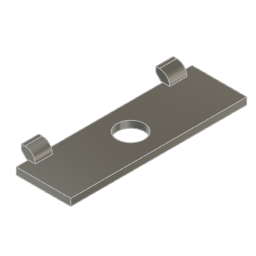
Mouse_ReplacementDoor (Autodesk Fusion 360 design; units mm, degrees)
Autodesk Fusion 360 part; units mm, degrees
sketch "Sketch1" plane through (0, 0, 0) normal (0, 0, 1) x (1, 0, 0)
  line L0 (0, 0) -> (15.8, 0)
  line L1 (15.8, 0) -> (15.8, 51)
  line L2 (15.8, 51) -> (0, 51)
  line L3 (0, 51) -> (0, 0)
  dimension "d1" = 15.8
  dimension "d2" = 51
  constraint horizontal L0
  constraint vertical L1
  constraint horizontal L2
  constraint vertical L3
  constraint coincident L0.start L3.end
  measures "d1" distance of L1.end L2.end
  measures "d2" distance of L0.end L1.end
extrude "Extrude1" add sketch "Sketch1" along normal blind 2
sketch "Sketch2" plane through (0, 0, 0) normal (0, 0, -1) x (1, 0, 0)
  line L0 (0, 0) -> (0, -51)
  line L1 (0, -51) -> (15.8, -51)
  line L2 (15.8, -51) -> (15.8, 0)
  line L3 (15.8, 0) -> (0, 0)
  circle A0 centre (7.6687, -25.5) radius 4
  dimension "d5" = 8
  measures "d5" diameter of A0
extrude "Extrude2" cut sketch "Sketch2" against normal blind 2 contours A0
sketch "Sketch3" plane through (0, 0, 2) normal (0, 0, 1) x (-1, 0, 0)
  line L0 (0, -51) -> (0, 0)
  line L1 (0, 0) -> (-15.8, 0)
  line L2 (-15.8, 0) -> (-15.8, -51)
  line L3 (-15.8, -51) -> (0, -51)
  line L4 (0, -3.5) -> (-2, -3.5)
  line L5 (-2, -3.5) -> (-2, -8.5)
  line L6 (-2, -8.5) -> (0, -8.5)
  line L7 (0, -8.5) -> (0, -3.5)
  line L8 (0, -42.5) -> (-2, -42.5)
  line L9 (-2, -42.5) -> (-2, -47.5)
  line L10 (-2, -47.5) -> (0, -47.5)
  line L11 (0, -47.5) -> (0, -42.5)
  circle A0 centre (-7.6687, -25.5) radius 4
  dimension "d8" = 3.5
  dimension "d9" = 42.5
  dimension "d10" = 2
  dimension "d11" = 2
  dimension "d12" = 5
  dimension "d13" = 5
  constraint horizontal L4
  constraint vertical L5
  constraint horizontal L6
  constraint vertical L7
  constraint coincident L0 L4.start
  constraint horizontal L8
  constraint vertical L9
  constraint horizontal L10
  constraint vertical L11
  constraint coincident L0 L8.start
  measures "d8" distance of L1 L4
  measures "d9" distance of L1 L8
  measures "d10" distance of L9.end L10.end
  measures "d11" distance of L5.end L6.end
  measures "d12" distance of L4.end L5.end
  measures "d13" distance of L8.end L9.end
extrude "Extrude3" add sketch "Sketch3" along normal blind 3 contours L0 L8 L9 L10 L11 | L0 L4 L5 L6 L7
sketch "Sketch4" plane through (0, 0, 0) normal (-1, 0, 0) x (0, -1, 0)
  line L0 (-51, 0) -> (0, 0)
  line L1 (0, 0) -> (0, 2)
  line L2 (0, 2) -> (-3.5, 2)
  line L3 (-3.5, 2) -> (-3.5, 5)
  line L4 (-3.5, 5) -> (-8.5, 5)
  line L5 (-8.5, 5) -> (-8.5, 2)
  line L6 (-8.5, 2) -> (-42.5, 2)
  line L7 (-42.5, 2) -> (-42.5, 5)
  line L8 (-42.5, 5) -> (-47.5, 5)
  line L9 (-47.5, 5) -> (-47.5, 2)
  line L10 (-47.5, 2) -> (-51, 2)
  line L11 (-51, 2) -> (-51, 0)
  line L12 (-47.5, 5) -> (-42.5, 5)
  line L13 (-42.5, 5) -> (-42.5, 2)
  line L14 (-42.5, 2) -> (-47.5, 2)
  line L15 (-47.5, 2) -> (-47.5, 5)
  line L16 (-8.5, 5) -> (-3.5, 5)
  line L17 (-3.5, 5) -> (-3.5, 2)
  line L18 (-3.5, 2) -> (-8.5, 2)
  line L19 (-8.5, 2) -> (-8.5, 5)
  constraint horizontal L12
  constraint vertical L13
  constraint horizontal L14
  constraint vertical L15
  constraint coincident L6.end L7.start
  constraint coincident L8.end L9.start
  constraint horizontal L16
  constraint vertical L17
  constraint horizontal L18
  constraint vertical L19
  constraint coincident L2.end L3.start
  constraint coincident L4.end L5.start
extrude "Extrude4" add sketch "Sketch4" along normal blind 2 contours L7 L8 L9 L12 L13 L14 L15 | L3 L4 L5 L16 L17 L18 L19
fillet "Fillet1" radius 3 1 edges at (2, 6, 5)
fillet "Fillet2" radius 3 1 edges at (2, 45, 5)
chamfer "Chamfer1" distance 1.5 angle 45 1 edges at (-2, 6, 2)
chamfer "Chamfer2" distance 1.5 angle 45 1 edges at (-2, 45, 2)
